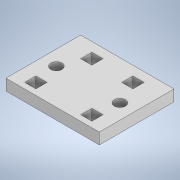
# Autodesk Inventor part: motorbase_3
Saved by Autodesk Inventor 2022 (Build 260153000, 153)
## iProperties
Created: 2023-04-18
Part Number: motorbase_3
Material: 一般
Document SubType Name: Modeling
Designer: Johnny Jou
Density: 1 g/cm^3
Appearance: 預設
Author: Johnny Jou
Autodesk Inventor part; units mm, degrees
ref_plane "YZ Plane" through (0, 0, 0) normal (1, 0, 0) x (0, 1, 0)
ref_plane "XZ Plane" through (0, 0, 0) normal (0, 1, 0) x (-1, 0, 0)
ref_plane "XY Plane" through (0, 0, 0) normal (0, 0, 1) x (1, 0, 0)
sketch "草圖1" plane through (0, 0, 0) normal (0, 1, 0) x (-1, 0, 0)
  line L0 (25, 0) -> (0, 0)
  line L1 (0, 0) -> (0, -20)
  line L2 (0, -20) -> (25, -20)
  line L3 (25, -20) -> (25, 0)
  line L4 (6.5, -14.5) -> (18.5, -14.5) construction
  line L5 (5.5, -17.5) -> (8.5, -17.5)
  line L6 (8.5, -17.5) -> (8.5, -14.5)
  line L7 (8.5, -14.5) -> (5.5, -14.5)
  line L8 (5.5, -14.5) -> (5.5, -17.5)
  line L9 (6.5, -4.5) -> (18.5, -4.5) construction
  line L10 (6.5, -4.5) -> (3.5, -4.5)
  line L11 (3.5, -4.5) -> (3.5, -1.5)
  line L12 (3.5, -1.5) -> (6.5, -1.5)
  line L13 (6.5, -1.5) -> (6.5, -4.5)
  line L14 (18.5, -4.5) -> (21.5, -4.5)
  line L15 (21.5, -4.5) -> (21.5, -1.5)
  line L16 (21.5, -1.5) -> (18.5, -1.5)
  line L17 (18.5, -1.5) -> (18.5, -4.5)
  line L18 (16.5, -17.5) -> (19.5, -17.5)
  line L19 (19.5, -17.5) -> (19.5, -14.5)
  line L20 (19.5, -14.5) -> (16.5, -14.5)
  line L21 (16.5, -14.5) -> (16.5, -17.5)
  circle A0 centre (4, -9.5) radius 1.5
  circle A1 centre (21, -9.5) radius 1.5
  point P0 (21.5, 16.3854)
  dimension "d0" = 25
  dimension "d1" = 20
  dimension "d2" = 3
  dimension "d3" = 3
  dimension "d4" = 0
  dimension "d5" = 10
  dimension "d6" = 3
  dimension "d7" = 3
  dimension "d8" = 3
  dimension "d9" = 3
  dimension "d10" = 3
  dimension "d11" = 3
  dimension "d12" = 3
  dimension "d13" = 5
  dimension "d14" = 5
  dimension "d15" = 8
  dimension "d16" = 2.5
  dimension "d17" = 3.5
  dimension "d18" = 12
  dimension "d19" = 2
  constraints: 44 end point, 10 parallel, 6 horizontal, 5 perpendicular, 2 centre point, 2 collinear, 1 coincident, 1 point on line
  measures "d0" distance of L1.end L2.end
  measures "d1" distance of L2.end L0.start
  measures "d2" distance of L7.end L5.start
  measures "d3" distance of L6.end L7.end
  measures "d4" distance between parallel lines of L4 L7
  measures "d5" distance between parallel lines of L4 L9
  measures "d6" distance of L11.start L12.start
  measures "d7" distance of L12.start L13.start
  measures "d8" distance of L21.end L18.end
  measures "d9" distance of L18.end L20.start
  measures "d10" distance of L9.end L14.end
  measures "d11" diameter of A0
  measures "d12" diameter of A1
  measures "d13" distance from line of L10 A0.centre
  measures "d14" distance from line of L14 A1.centre
  measures "d15" distance between parallel lines of L21 L6
  measures "d16" distance between parallel lines of L2 L18
  measures "d17" distance between parallel lines of L3 L15
  measures "d18" distance between parallel lines of L13 L17
  measures "d19" distance between parallel lines of L21 L17
extrude "擠出1" add sketch "草圖1" along normal blind 3
